Autodesk Fusion 360 part; units mm, degrees
(part 5 of 5)
  line L1149 (-30.3799, -38.9795, 1210.5243) -> (-23.832, -44.0828, 1211.5804) construction
  line L1150 (-23.832, -44.0828, 1211.5804) -> (-15.9786, -47.4967, 1212.6365) construction
  line L1151 (-15.9786, -47.4967, 1212.6365) -> (-7.7804, -48.8037, 1213.6926) construction
  line L1152 (-7.7804, -48.8037, 1213.6926) -> (0.4171, -50.1106, 1214.7486) construction
  line L1153 (0.4171, -50.1106, 1214.7486) -> (8.942, -49.3081, 1215.8046) construction
  line L1154 (8.942, -49.3081, 1215.8046) -> (16.7516, -46.4943, 1216.8606) construction
  line L1155 (16.7516, -46.4943, 1216.8606) -> (24.5605, -43.6808, 1217.9165) construction
  line L1156 (24.5605, -43.6808, 1217.9165) -> (31.6378, -38.8624, 1218.9725) construction
  line L1157 (31.6378, -38.8624, 1218.9725) -> (37.1178, -32.6282, 1220.0284) construction
  line L1158 (37.1178, -32.6282, 1220.0284) -> (42.5975, -26.3946, 1221.0842) construction
  line L1159 (42.5975, -26.3946, 1221.0842) -> (46.4686, -18.7588, 1222.1401) construction
  line L1160 (46.4686, -18.7588, 1222.1401) -> (48.2579, -10.6544, 1223.1959) construction
  line L1161 (48.2579, -10.6544, 1223.1959) -> (50.047, -2.5506, 1224.2516) construction
  line L1162 (50.047, -2.5506, 1224.2516) -> (49.7509, 6.0046, 1225.3074) construction
  line L1163 (49.7509, 6.0046, 1225.3074) -> (47.4058, 13.9653, 1226.3631) construction
  line L1164 (47.4058, 13.9653, 1226.3631) -> (45.0608, 21.9253, 1227.4188) construction
  line L1165 (45.0608, 21.9253, 1227.4188) -> (40.6721, 29.2741, 1228.4744) construction
  line L1166 (40.6721, 29.2741, 1228.4744) -> (34.7761, 35.1135, 1229.5301) construction
  line L1167 (34.7761, 35.1135, 1229.5301) -> (28.8806, 40.9524, 1230.5857) construction
  line L1168 (28.8806, 40.9524, 1230.5857) -> (21.4905, 45.2697, 1231.6412) construction
  line L1169 (21.4905, 45.2697, 1231.6412) -> (13.509, 47.5378, 1232.6968) construction
  line L1170 (13.509, 47.5378, 1232.6968) -> (5.528, 49.8058, 1233.7523) construction
  line L1171 (5.528, 49.8058, 1233.7523) -> (-3.0273, 50.0201, 1234.8078) construction
  line L1172 (-3.0273, 50.0201, 1234.8078) -> (-11.1118, 48.1546, 1235.8633) construction
  line L1173 (-11.1118, 48.1546, 1235.8633) -> (-19.1956, 46.2892, 1236.9187) construction
  line L1174 (-19.1956, 46.2892, 1236.9187) -> (-26.7915, 42.3483, 1237.9741) construction
  line L1175 (-26.7915, 42.3483, 1237.9741) -> (-32.9714, 36.8134, 1239.0295) construction
  line L1176 (-32.9714, 36.8134, 1239.0295) -> (-39.1508, 31.2788, 1240.0848) construction
  line L1177 (-39.1508, 31.2788, 1240.0848) -> (-43.9015, 24.1622, 1241.1401) construction
  line L1178 (-43.9015, 24.1622, 1241.1401) -> (-46.6431, 16.3327, 1242.1954) construction
  line L1179 (-46.6431, 16.3327, 1242.1954) -> (-49.3845, 8.5039, 1243.2507) construction
  line L1180 (-49.3845, 8.5039, 1243.2507) -> (-50.1113, -0.0211, 1244.3059) construction
  line L1181 (-50.1113, -0.0211, 1244.3059) -> (-48.7348, -8.201, 1245.3611) construction
  line L1182 (-48.7348, -8.201, 1245.3611) -> (-47.3584, -16.3803, 1246.4163) construction
  line L1183 (-47.3584, -16.3803, 1246.4163) -> (-43.8819, -24.1973, 1247.4714) construction
  line L1184 (-43.8819, -24.1973, 1247.4714) -> (-38.7299, -30.6974, 1248.5266) construction
  line L1185 (-38.7299, -30.6974, 1248.5266) -> (-33.5783, -37.1971, 1249.5817) construction
  line L1186 (-33.5783, -37.1971, 1249.5817) -> (-26.7622, -42.3663, 1250.6367) construction
  line L1187 (-26.7622, -42.3663, 1250.6367) -> (-19.114, -45.574, 1251.6918) construction
  line L1188 (-19.114, -45.574, 1251.6918) -> (-11.4664, -48.7815, 1252.7468) construction
  line L1189 (-11.4664, -48.7815, 1252.7468) -> (-3.0029, -50.0209, 1253.8018) construction
  line L1190 (-3.0029, -50.0209, 1253.8018) -> (5.2434, -49.1411, 1254.8568) construction
  line L1191 (5.2434, -49.1411, 1254.8568) -> (13.4889, -48.2613, 1255.9117) construction
  line L1192 (13.4889, -48.2613, 1255.9117) -> (21.4998, -45.2643, 1256.9666) construction
  line L1193 (21.4998, -45.2643, 1256.9666) -> (28.2982, -40.516, 1258.0215) construction
  line L1194 (28.2982, -40.516, 1258.0215) -> (35.096, -35.7681, 1259.0764) construction
  line L1195 (35.096, -35.7681, 1259.0764) -> (40.6672, -29.2792, 1260.1312) construction
  line L1196 (40.6672, -29.2792, 1260.1312) -> (44.3317, -21.8411, 1261.186) construction
  line L1197 (44.3317, -21.8411, 1261.186) -> (47.996, -14.4036, 1262.2408) construction
  line L1198 (47.996, -14.4036, 1262.2408) -> (49.7462, -6.0329, 1263.2955) construction
  line L1199 (49.7462, -6.0329, 1263.2955) -> (49.3688, 2.2497, 1264.3503) construction
  line L1200 (49.3688, 2.2497, 1264.3503) -> (48.9914, 10.5317, 1265.405) construction
  line L1201 (48.9914, 10.5317, 1265.405) -> (46.4874, 18.708, 1266.4597) construction
  line L1202 (46.4874, 18.708, 1266.4597) -> (42.1625, 25.781, 1267.5143) construction
  line L1203 (42.1625, 25.781, 1267.5143) -> (37.8378, 32.8536, 1268.5689) construction
  line L1204 (37.8378, 32.8536, 1268.5689) -> (31.7016, 38.8081, 1269.6235) construction
  line L1205 (31.7016, 38.8081, 1269.6235) -> (24.5023, 42.9182, 1270.6781) construction
  line L1206 (24.5023, 42.9182, 1270.6781) -> (17.3034, 47.0281, 1271.7327) construction
  line L1207 (17.3034, 47.0281, 1271.7327) -> (9.0569, 49.2851, 1272.7872) construction
  line L1208 (9.0569, 49.2851, 1272.7872) -> (0.7686, 49.414, 1273.8417) construction
  line L1209 (0.7686, 49.414, 1273.8417) -> (-7.5192, 49.5429, 1274.8962) construction
  line L1210 (-7.5192, 49.5429, 1274.8962) -> (-15.8313, 47.5438, 1275.9506) construction
  line L1211 (-15.8313, 47.5438, 1275.9506) -> (-23.1541, 43.6603, 1277.0051) construction
  line L1212 (-23.1541, 43.6603, 1277.0051) -> (-30.4764, 39.7772, 1278.0595) construction
  line L1213 (-30.4764, 39.7772, 1278.0595) -> (-36.7939, 34.0182, 1279.1138) construction
  line L1214 (-36.7939, 34.0182, 1279.1138) -> (-41.3365, 27.0857, 1280.1682) construction
  line L1215 (-41.3365, 27.0857, 1280.1682) -> (-45.8787, 20.1536, 1281.2225) construction
  line L1216 (-45.8787, 20.1536, 1281.2225) -> (-48.6365, 12.0628, 1282.2768) construction
  line L1217 (-48.6365, 12.0628, 1282.2768) -> (-49.2737, 3.7997, 1283.3311) construction
  line L1218 (-49.2737, 3.7997, 1283.3311) -> (-49.9109, -4.4628, 1284.3854) construction
  line L1219 (-49.9109, -4.4628, 1284.3854) -> (-48.4264, -12.8802, 1285.4396) construction
  line L1220 (-48.4264, -12.8802, 1285.4396) -> (-45.0012, -20.4263, 1286.4938) construction
  line L1221 (-45.0012, -20.4263, 1286.4938) -> (-41.5762, -27.9718, 1287.548) construction
  line L1222 (-41.5762, -27.9718, 1287.548) -> (-36.218, -34.6303, 1288.6022) construction
  line L1223 (-36.218, -34.6303, 1288.6022) -> (-29.5797, -39.5901, 1289.6563) construction
  line L1224 (-29.5797, -39.5901, 1289.6563) -> (-22.9419, -44.5496, 1290.7104) construction
  line L1225 (-22.9419, -44.5496, 1290.7104) -> (-15.0381, -47.8001, 1291.7645) construction
  line L1226 (-15.0381, -47.8001, 1291.7645) -> (-6.8317, -48.9455, 1292.8186) construction
  line L1227 (-6.8317, -48.9455, 1292.8186) -> (1.3741, -50.0909, 1293.8726) construction
  line L1228 (1.3741, -50.0909, 1293.8726) -> (9.8653, -49.129, 1294.9267) construction
  line L1229 (9.8653, -49.129, 1294.9267) -> (17.607, -46.1771, 1295.9807) construction
  line L1230 (17.607, -46.1771, 1295.9807) -> (25.3483, -43.2255, 1297.0346) construction
  line L1231 (25.3483, -43.2255, 1297.0346) -> (32.3239, -38.2903, 1298.0886) construction
  line L1232 (32.3239, -38.2903, 1298.0886) -> (37.6838, -31.9729, 1299.1426) construction
  line L1233 (37.6838, -31.9729, 1299.1426) -> (43.0435, -25.6559, 1300.1964) construction
  line L1234 (43.0435, -25.6559, 1300.1964) -> (46.7765, -17.9702, 1301.2503) construction
  line L1235 (46.7765, -17.9702, 1301.2503) -> (48.428, -9.8521, 1302.3042) construction
  line L1236 (48.428, -9.8521, 1302.3042) -> (50.0794, -1.7346, 1303.358) construction
  line L1237 (50.0794, -1.7346, 1303.358) -> (49.6462, 6.7981, 1304.4119) construction
  line L1238 (49.6462, 6.7981, 1304.4119) -> (47.181, 14.7066, 1305.4657) construction
  line L1239 (47.181, 14.7066, 1305.4657) -> (44.7161, 22.6147, 1306.5194) construction
  line L1240 (44.7161, 22.6147, 1306.5194) -> (40.2246, 29.8819, 1307.5732) construction
  line L1241 (40.2246, 29.8819, 1307.5732) -> (34.2538, 35.6232, 1308.6269) construction
  line L1242 (34.2538, 35.6232, 1308.6269) -> (28.2834, 41.3641, 1309.6806) construction
  line L1243 (28.2834, 41.3641, 1309.6806) -> (20.8463, 45.5672, 1310.7343) construction
  line L1244 (20.8463, 45.5672, 1310.7343) -> (12.8484, 47.7206, 1311.788) construction
  line L1245 (12.8484, 47.7206, 1311.788) -> (4.8509, 49.8738, 1312.8416) construction
  line L1246 (4.8509, 49.8738, 1312.8416) -> (-3.6905, 49.9731, 1313.8953) construction
  line L1247 (-3.6905, 49.9731, 1313.8953) -> (-11.7359, 48.0063, 1314.9489) construction
  line L1248 (-11.7359, 48.0063, 1314.9489) -> (-19.7807, 46.0396, 1316.0024) construction
  line L1249 (-19.7807, 46.0396, 1316.0024) -> (-27.3126, 42.0112, 1317.056) construction
  line L1250 (-27.3126, 42.0112, 1317.056) -> (-33.4145, 36.4117, 1318.1096) construction
  line L1251 (-33.4145, 36.4117, 1318.1096) -> (-39.5159, 30.8124, 1319.1631) construction
  line L1252 (-39.5159, 30.8124, 1319.1631) -> (-44.1747, 23.654, 1320.2166) construction
  line L1253 (-44.1747, 23.654, 1320.2166) -> (-46.8236, 15.8078, 1321.2701) construction
  line L1254 (-46.8236, 15.8078, 1321.2701) -> (-49.4724, 7.962, 1322.3235) construction
  line L1255 (-49.4724, 7.962, 1322.3235) -> (-50.1059, -0.5549, 1323.3769) construction
  line L1256 (-50.1059, -0.5549, 1323.3769) -> (-48.6471, -8.7061, 1324.4304) construction
  line L1257 (-48.6471, -8.7061, 1324.4304) -> (-47.1884, -16.8569, 1325.4837) construction
  line L1258 (-47.1884, -16.8569, 1325.4837) -> (-43.6407, -24.625, 1326.5371) construction
  line L1259 (-43.6407, -24.625, 1326.5371) -> (-38.4357, -31.0649, 1327.5905) construction
  line L1260 (-38.4357, -31.0649, 1327.5905) -> (-33.2311, -37.5045, 1328.6438) construction
  line L1261 (-33.2311, -37.5045, 1328.6438) -> (-26.3804, -42.6024, 1329.6971) construction
  line L1262 (-26.3804, -42.6024, 1329.6971) -> (-18.7174, -45.7383, 1330.7504) construction
  line L1263 (-18.7174, -45.7383, 1330.7504) -> (-11.0549, -48.8741, 1331.8037) construction
  line L1264 (-11.0549, -48.8741, 1331.8037) -> (-2.5962, -50.0414, 1332.8569) construction
  line L1265 (-2.5962, -50.0414, 1332.8569) -> (5.6293, -49.0983, 1333.9102) construction
  line L1266 (5.6293, -49.0983, 1333.9102) -> (13.8543, -48.1553, 1334.9634) construction
  line L1267 (13.8543, -48.1553, 1334.9634) -> (21.8289, -45.1041, 1336.0166) construction
  line L1268 (21.8289, -45.1041, 1336.0166) -> (28.5826, -40.3159, 1337.0698) construction
  line L1269 (28.5826, -40.3159, 1337.0698) -> (35.336, -35.5279, 1338.1229) construction
  line L1270 (35.336, -35.5279, 1338.1229) -> (40.8546, -29.0133, 1339.1761) construction
  line L1271 (40.8546, -29.0133, 1339.1761) -> (44.4669, -21.5645, 1340.2292) construction
  line L1272 (44.4669, -21.5645, 1340.2292) -> (48.079, -14.1162, 1341.2823) construction
  line L1273 (48.079, -14.1162, 1341.2823) -> (49.7776, -5.7495, 1342.3354) construction
  line L1274 (49.7776, -5.7495, 1342.3354) -> (49.3558, 2.5177, 1343.3884) construction
  line L1275 (49.3558, 2.5177, 1343.3884) -> (48.9341, 10.7846, 1344.4415) construction
  line L1276 (48.9341, 10.7846, 1344.4415) -> (46.3933, 18.9346, 1345.4945) construction
  line L1277 (46.3933, 18.9346, 1345.4945) -> (42.0424, 25.9764, 1346.5475) construction
  line L1278 (42.0424, 25.9764, 1346.5475) -> (37.6917, 33.0179, 1347.6005) construction
  line L1279 (37.6917, 33.0179, 1347.6005) -> (31.5403, 38.9365, 1348.6534) construction
  line L1280 (31.5403, 38.9365, 1348.6534) -> (24.3364, 43.0125, 1349.7064) construction
  line L1281 (24.3364, 43.0125, 1349.7064) -> (16.8312, 47.2589, 1350.8034) construction
  line L1282 (16.8312, 47.2589, 1350.8034) -> (8.1992, 49.4921, 1351.9004) construction
  line L1283 (8.1992, 49.4921, 1351.9004) -> (-0.4236, 49.4182, 1352.9974) construction
  line L1284 (-0.4236, 49.4182, 1352.9974) -> (-8.9118, 49.3454, 1354.0772) construction
  line L1285 (-8.9118, 49.3454, 1354.0772) -> (-17.3709, 47.0387, 1355.1571) construction
  line L1286 (-17.3709, 47.0387, 1355.1571) -> (-24.721, 42.7926, 1356.2369) construction
  line L1287 (-24.721, 42.7926, 1356.2369) -> (-31.9563, 38.6129, 1357.2999) construction
  line L1288 (-31.9563, 38.6129, 1357.2999) -> (-38.1014, 32.5643, 1358.3629) construction
  line L1289 (-38.1014, 32.5643, 1358.3629) -> (-42.3954, 25.3962, 1359.4259) construction
  line L1290 (-42.3954, 25.3962, 1359.4259) -> (-46.668, 18.2637, 1360.4836) construction
  line L1291 (-46.668, 18.2637, 1360.4836) -> (-49.0989, 10.0382, 1361.5413) construction
  line L1292 (-49.0989, 10.0382, 1361.5413) -> (-49.3897, 1.729, 1362.599) construction
  line L1293 (-49.3897, 1.729, 1362.599) -> (-49.6806, -6.5787, 1363.6565) construction
  line L1294 (-49.6806, -6.5787, 1363.6565) -> (-47.8316, -14.9523, 1364.714) construction
  line L1295 (-47.8316, -14.9523, 1364.714) -> (-44.0697, -22.3651, 1365.7715) construction
  line L1296 (-44.0697, -22.3651, 1365.7715) -> (-40.3085, -29.7764, 1366.8288) construction
  line L1297 (-40.3085, -29.7764, 1366.8288) -> (-34.6431, -36.2115, 1367.8861) construction
  line L1298 (-34.6431, -36.2115, 1367.8861) -> (-27.7679, -40.8813, 1368.9434) construction
  line L1299 (-27.7679, -40.8813, 1368.9434) -> (-20.8941, -45.5502, 1370.0005) construction
  line L1300 (-20.8941, -45.5502, 1370.0005) -> (-12.8257, -48.4447, 1371.0576) construction
  line L1301 (-12.8257, -48.4447, 1371.0576) -> (-4.5515, -49.21, 1372.1147) construction
  line L1302 (-4.5515, -49.21, 1372.1147) -> (3.7212, -49.9751, 1373.1716) construction
  line L1303 (3.7212, -49.9751, 1373.1716) -> (12.182, -48.6103, 1374.2285) construction
  line L1304 (12.182, -48.6103, 1374.2285) -> (19.7944, -45.2826, 1375.2853) construction
  line L1305 (19.7944, -45.2826, 1375.2853) -> (27.4055, -41.9556, 1376.342) construction
  line L1306 (27.4055, -41.9556, 1376.342) -> (34.1523, -36.6736, 1377.3987) construction
  line L1307 (34.1523, -36.6736, 1377.3987) -> (39.2087, -30.0835, 1378.4555) construction
  line L1308 (39.2087, -30.0835, 1378.4555) -> (44.2642, -23.4945, 1379.512) construction
  line L1309 (44.2642, -23.4945, 1379.512) -> (47.6191, -15.6119, 1380.5685) construction
  line L1310 (47.6191, -15.6119, 1380.5685) -> (48.8627, -7.4006, 1381.625) construction
  line L1311 (48.8627, -7.4006, 1381.625) -> (50.1062, 0.8092, 1382.6813) construction
  line L1312 (50.1062, 0.8092, 1382.6813) -> (49.2365, 9.3302, 1383.7376) construction
  line L1313 (49.2365, 9.3302, 1383.7376) -> (46.3601, 17.1195, 1384.7939) construction
  line L1314 (46.3601, 17.1195, 1384.7939) -> (43.4842, 24.9075, 1385.8501) construction
  line L1315 (43.4842, 24.9075, 1385.8501) -> (38.6084, 31.9476, 1386.9062) construction
  line L1316 (38.6084, 31.9476, 1386.9062) -> (32.3292, 37.3786, 1387.9624) construction
  line L1317 (32.3292, 37.3786, 1387.9624) -> (26.0511, 42.8086, 1389.0183) construction
  line L1318 (26.0511, 42.8086, 1389.0183) -> (18.3833, 46.6185, 1390.0743) construction
  line L1319 (18.3833, 46.6185, 1390.0743) -> (10.2637, 48.3424, 1391.1302) construction
  line L1320 (10.2637, 48.3424, 1391.1302) -> (2.1455, 50.0661, 1392.186) construction
  line L1321 (2.1455, 50.0661, 1392.186) -> (-6.4073, 49.7007, 1393.2418) construction
  line L1322 (-6.4073, 49.7007, 1393.2418) -> (-14.349, 47.291, 1394.2976) construction
  line L1323 (-14.349, 47.291, 1394.2976) -> (-22.2894, 44.8818, 1395.3532) construction
  line L1324 (-22.2894, 44.8818, 1395.3532) -> (-29.6021, 40.434, 1396.4088) construction
  line L1325 (-29.6021, 40.434, 1396.4088) -> (-35.3933, 34.4913, 1397.4644) construction
  line L1326 (-35.3933, 34.4913, 1397.4644) -> (-41.1836, 28.5496, 1398.5198) construction
  line L1327 (-41.1836, 28.5496, 1398.5198) -> (-45.4407, 21.126, 1399.5753) construction
  line L1328 (-45.4407, 21.126, 1399.5753) -> (-47.6446, 13.1275, 1400.6307) construction
  line L1329 (-47.6446, 13.1275, 1400.6307) -> (-49.848, 5.1303, 1401.686) construction
  line L1330 (-49.848, 5.1303, 1401.686) -> (-49.9942, -3.4246, 1402.7412) construction
  line L1331 (-49.9942, -3.4246, 1402.7412) -> (-48.0652, -11.4924, 1403.7965) construction
  line L1332 (-48.0652, -11.4924, 1403.7965) -> (-46.1365, -19.5589, 1404.8516) construction
  line L1333 (-46.1365, -19.5589, 1404.8516) -> (-42.1374, -27.1214, 1405.9067) construction
  line L1334 (-42.1374, -27.1214, 1405.9067) -> (-36.5561, -33.2564, 1406.9618) construction
  line L1335 (-36.5561, -33.2564, 1406.9618) -> (-30.9757, -39.3905, 1408.0168) construction
  line L1336 (-30.9757, -39.3905, 1408.0168) -> (-23.8255, -44.0846, 1409.0717) construction
  line L1337 (-23.8255, -44.0846, 1409.0717) -> (-15.9782, -46.7657, 1410.1266) construction
  line L1338 (-15.9782, -46.7657, 1410.1266) -> (-8.1321, -49.4465, 1411.1814) construction
  line L1339 (-8.1321, -49.4465, 1411.1814) -> (0.3942, -50.1092, 1412.2362) construction
  line L1340 (0.3942, -50.1092, 1412.2362) -> (8.5603, -48.673, 1413.291) construction
  line L1341 (8.5603, -48.673, 1413.291) -> (16.7251, -47.237, 1414.3456) construction
  line L1342 (16.7251, -47.237, 1414.3456) -> (24.5126, -43.7058, 1415.4003) construction
  line L1343 (24.5126, -43.7058, 1415.4003) -> (30.9727, -38.5101, 1416.4549) construction
  line L1344 (30.9727, -38.5101, 1416.4549) -> (37.4319, -33.3152, 1417.5094) construction
  line L1345 (37.4319, -33.3152, 1417.5094) -> (42.5503, -26.4673, 1418.5639) construction
  line L1346 (42.5503, -26.4673, 1418.5639) -> (45.7038, -18.8015, 1419.6184) construction
  line L1347 (45.7038, -18.8015, 1419.6184) -> (48.8569, -11.1369, 1420.6727) construction
  line L1348 (48.8569, -11.1369, 1420.6727) -> (50.0389, -2.6709, 1421.727) construction
  line L1349 (50.0389, -2.6709, 1421.727) -> (49.1058, 5.5643, 1422.7814) construction
  line L1350 (49.1058, 5.5643, 1422.7814) -> (48.1727, 13.7983, 1423.8356) construction
  line L1351 (48.1727, 13.7983, 1423.8356) -> (45.1271, 21.7842, 1424.8897) construction
  line L1352 (45.1271, 21.7842, 1424.8897) -> (40.3401, 28.5484, 1425.9439) construction
  line L1353 (40.3401, 28.5484, 1425.9439) -> (35.5538, 35.3117, 1426.998) construction
  line L1354 (35.5538, 35.3117, 1426.998) -> (29.0366, 40.8395, 1428.052) construction
  line L1355 (29.0366, 40.8395, 1428.052) -> (21.5829, 44.458, 1429.1061) construction
  line L1356 (21.5829, 44.458, 1429.1061) -> (14.1302, 48.0761, 1430.16) construction
  line L1357 (14.1302, 48.0761, 1430.16) -> (5.7568, 49.7778, 1431.2139) construction
  line L1358 (5.7568, 49.7778, 1431.2139) -> (-2.517, 49.3559, 1432.2678) construction
  line L1359 (-2.517, 49.3559, 1432.2678) -> (-10.7897, 48.934, 1433.3216) construction
  line L1360 (-10.7897, 48.934, 1433.3216) -> (-18.9455, 46.3899, 1434.3754) construction
  line L1361 (-18.9455, 46.3899, 1434.3754) -> (-25.9909, 42.0334, 1435.4292) construction
  line L1362 (-25.9909, 42.0334, 1435.4292) -> (-33.0354, 37.6775, 1436.4828) construction
  line L1363 (-33.0354, 37.6775, 1436.4828) -> (-38.955, 31.5189, 1437.5365) construction
  line L1364 (-38.955, 31.5189, 1437.5365) -> (-43.0288, 24.3076, 1438.5901) construction
  line L1365 (-43.0288, 24.3076, 1438.5901) -> (-47.1021, 17.0971, 1439.6436) construction
  line L1366 (-47.1021, 17.0971, 1439.6436) -> (-49.3215, 8.8493, 1440.6972) construction
  line L1367 (-49.3215, 8.8493, 1440.6972) -> (-49.4167, 0.5684, 1441.7507) construction
  line L1368 (-49.4167, 0.5684, 1441.7507) -> (-49.512, -7.7116, 1442.8041) construction
  line L1369 (-49.512, -7.7116, 1442.8041) -> (-47.4834, -16.0072, 1443.8575) construction
  line L1370 (-47.4834, -16.0072, 1443.8575) -> (-43.5779, -23.3089, 1444.9109) construction
  line L1371 (-43.5779, -23.3089, 1444.9109) -> (-39.6729, -30.6097, 1445.9642) construction
  line L1372 (-39.6729, -30.6097, 1445.9642) -> (-33.8996, -36.9013, 1447.0174) construction
  line L1373 (-33.8996, -36.9013, 1447.0174) -> (-26.9606, -41.4181, 1448.0707) construction
  line L1374 (-26.9606, -41.4181, 1448.0707) -> (-20.0224, -45.9345, 1449.1239) construction
  line L1375 (-20.0224, -45.9345, 1449.1239) -> (-11.9334, -48.6669, 1450.177) construction
  line L1376 (-11.9334, -48.6669, 1450.177) -> (-3.6777, -49.283, 1451.2302) construction
  line L1377 (-3.6777, -49.283, 1451.2302) -> (4.5771, -49.899, 1452.2833) construction
  line L1378 (4.5771, -49.899, 1452.2833) -> (12.9811, -48.3978, 1453.3363) construction
  line L1379 (12.9811, -48.3978, 1453.3363) -> (20.5122, -44.9621, 1454.3893) construction
  line L1380 (20.5122, -44.9621, 1454.3893) -> (28.4043, -41.3616, 1455.4929) construction
  line L1381 (28.4043, -41.3616, 1455.4929) -> (35.3172, -35.641, 1456.5964) construction
  line L1382 (35.3172, -35.641, 1456.5964) -> (40.3306, -28.5619, 1457.7) construction
  line L1383 (40.3306, -28.5619, 1457.7) -> (45.1873, -21.7039, 1458.769) construction
  line L1384 (45.1873, -21.7039, 1458.769) -> (48.2525, -13.5887, 1459.8381) construction
  line L1385 (48.2525, -13.5887, 1459.8381) -> (49.1422, -5.2323, 1460.9071) construction
  line L1386 (49.1422, -5.2323, 1460.9071) -> (50.0224, 3.0342, 1461.9647) construction
  line L1387 (50.0224, 3.0342, 1461.9647) -> (48.7726, 11.5186, 1463.0223) construction
  line L1388 (48.7726, 11.5186, 1463.0223) -> (45.5462, 19.1803, 1464.0798) construction
  line L1389 (45.5462, 19.1803, 1464.0798) -> (42.3209, 26.839, 1465.137) construction
  line L1390 (42.3209, 26.839, 1465.137) -> (37.1275, 33.6592, 1466.1942) construction
  line L1391 (37.1275, 33.6592, 1466.1942) -> (30.6023, 38.8051, 1467.2513) construction
  line L1392 (30.6023, 38.8051, 1467.2513) -> (24.0796, 43.949, 1468.3081) construction
  line L1393 (24.0796, 43.949, 1468.3081) -> (16.2401, 47.4089, 1469.3649) construction
  line L1394 (16.2401, 47.4089, 1469.3649) -> (8.0439, 48.761, 1470.4216) construction
  line L1395 (8.0439, 48.761, 1470.4216) -> (-0.1494, 50.1126, 1471.478) construction
  line L1396 (-0.1494, 50.1126, 1471.478) -> (-8.6816, 49.3551, 1472.5344) construction
  line L1397 (-8.6816, 49.3551, 1472.5344) -> (-16.5086, 46.5811, 1473.5908) construction
  line L1398 (-16.5086, 46.5811, 1473.5908) -> (-24.3328, 43.8082, 1474.6468) construction
  line L1399 (-24.3328, 43.8082, 1474.6468) -> (-31.4357, 39.0261, 1475.7028) construction
  line L1400 (-31.4357, 39.0261, 1475.7028) -> (-36.9485, 32.8199, 1476.7589) construction
  line L1401 (-36.9485, 32.8199, 1476.7589) -> (-42.4594, 26.6157, 1477.8145) construction
  line L1402 (-42.4594, 26.6157, 1477.8145) -> (-46.3696, 19.0014, 1478.8702) construction
  line L1403 (-46.3696, 19.0014, 1478.8702) -> (-48.2012, 10.9078, 1479.9259) construction
  line L1404 (-48.2012, 10.9078, 1479.9259) -> (-50.0322, 2.8167, 1480.9812) construction
  line L1405 (-50.0322, 2.8167, 1480.9812) -> (-49.782, -5.7363, 1482.0365) construction
  line L1406 (-49.782, -5.7363, 1482.0365) -> (-47.4812, -13.7065, 1483.0918) construction
  line L1407 (-47.4812, -13.7065, 1483.0918) -> (-45.1812, -21.6742, 1484.1468) construction
  line L1408 (-45.1812, -21.6742, 1484.1468) -> (-40.8367, -29.0427, 1485.2018) construction
  line L1409 (-40.8367, -29.0427, 1485.2018) -> (-34.9781, -34.9123, 1486.2568) construction
  line L1410 (-34.9781, -34.9123, 1486.2568) -> (-29.1213, -40.7802, 1487.3115) construction
  line L1411 (-29.1213, -40.7802, 1487.3115) -> (-21.7637, -45.1377, 1488.3662) construction
  line L1412 (-21.7637, -45.1377, 1488.3662) -> (-13.803, -47.4533, 1489.4209) construction
  line L1413 (-13.803, -47.4533, 1489.4209) -> (-5.8446, -49.7682, 1490.4753) construction
  line L1414 (-5.8446, -49.7682, 1490.4753) -> (2.6998, -50.0374, 1491.5297) construction
  line L1415 (2.6998, -50.0374, 1491.5297) -> (10.7882, -48.2281, 1492.584) construction
  line L1416 (10.7882, -48.2281, 1492.584) -> (18.8743, -46.4193, 1493.6381) construction
  line L1417 (18.8743, -46.4193, 1493.6381) -> (26.4877, -42.537, 1494.6922) construction
  line L1418 (26.4877, -42.537, 1494.6922) -> (32.7004, -37.0543, 1495.7463) construction
  line L1419 (32.7004, -37.0543, 1495.7463) -> (38.9115, -31.573, 1496.8002) construction
  line L1420 (38.9115, -31.573, 1496.8002) -> (43.7096, -24.5037, 1497.854) construction
  line L1421 (43.7096, -24.5037, 1497.854) -> (46.5101, -16.7076, 1498.9078) construction
  line L1422 (46.5101, -16.7076, 1498.9078) -> (49.31, -8.9134, 1499.9614) construction
  line L1423 (49.31, -8.9134, 1499.9614) -> (50.1075, -0.4092, 1501.015) construction
  line L1424 (50.1075, -0.4092, 1501.015) -> (48.8054, 7.7697, 1502.0685) construction
  line L1425 (48.8054, 7.7697, 1502.0685) -> (47.5037, 15.9466, 1503.1219) construction
  line L1426 (47.5037, 15.9466, 1503.1219) -> (44.1062, 23.781, 1504.1752) construction
  line L1427 (44.1062, 23.781, 1504.1752) -> (39.0264, 30.3195, 1505.2285) construction
  line L1428 (39.0264, 30.3195, 1505.2285) -> (33.9478, 36.8566, 1506.2816) construction
  line L1429 (33.9478, 36.8566, 1506.2816) -> (27.1983, 42.0846, 1507.3347) construction
  line L1430 (27.1983, 42.0846, 1507.3347) -> (19.5991, 45.3675, 1508.3877) construction
  line L1431 (19.5991, 45.3675, 1508.3877) -> (11.7904, 48.7409, 1509.4699) construction
  line L1432 (11.7904, 48.7409, 1509.4699) -> (3.1011, 50.0507, 1510.552) construction
  line L1433 (3.1011, 50.0507, 1510.552) -> (-5.355, 49.129, 1511.6341) construction
  line L1434 (-5.355, 49.129, 1511.6341) -> (-13.6173, 48.2284, 1512.6914) construction
  line L1435 (-13.6173, 48.2284, 1512.6914) -> (-21.6389, 45.2014, 1513.7487) construction
  line L1436 (-21.6389, 45.2014, 1513.7487) -> (-28.4364, 40.4191, 1514.806) construction
  line L1437 (-28.4364, 40.4191, 1514.806) -> (-35.2289, 35.6404, 1515.8625) construction
  line L1438 (-35.2289, 35.6404, 1515.8625) -> (-40.7846, 29.1192, 1516.919) construction
  line L1439 (-40.7846, 29.1192, 1516.919) -> (-44.4235, 21.6538, 1517.9756) construction
  line L1440 (-44.4235, 21.6538, 1517.9756) -> (-48.06, 14.1935, 1519.0314) construction
  line L1441 (-48.06, 14.1935, 1519.0314) -> (-49.7745, 5.8063, 1520.0872) construction
  line L1442 (-49.7745, 5.8063, 1520.0872) -> (-49.3576, -2.4825, 1521.1429) construction
  line L1443 (-49.3576, -2.4825, 1521.1429) -> (-48.941, -10.766, 1522.1981) construction
  line L1444 (-48.941, -10.766, 1522.1981) -> (-46.3965, -18.9338, 1523.2532) construction
  line L1445 (-46.3965, -18.9338, 1523.2532) -> (-42.035, -25.9883, 1524.3083) construction
  line L1446 (-42.035, -25.9883, 1524.3083) -> (-37.6761, -33.0388, 1525.3628) construction
  line L1447 (-37.6761, -33.0388, 1525.3628) -> (-31.5114, -38.9625, 1526.4173) construction
  line L1448 (-31.5114, -38.9625, 1526.4173) -> (-24.2929, -43.0371, 1527.4718) construction
  line L1449 (-24.2929, -43.0371, 1527.4718) -> (-17.0783, -47.1095, 1528.5257) construction
  line L1450 (-17.0783, -47.1095, 1528.5257) -> (-8.8262, -49.3262, 1529.5796) construction
  line L1451 (-8.8262, -49.3262, 1529.5796) -> (-0.5421, -49.417, 1530.6335) construction
  line L1452 (-0.5421, -49.417, 1530.6335) -> (7.738, -49.5079, 1531.6869) construction
  line L1453 (7.738, -49.5079, 1531.6869) -> (16.0326, -47.4748, 1532.7404) construction
  line L1454 (16.0326, -47.4748, 1532.7404) -> (23.3322, -43.5654, 1533.7938) construction
  line L1455 (23.3322, -43.5654, 1533.7938) -> (30.9937, -39.4621, 1534.8994) construction
  line L1456 (30.9937, -39.4621, 1534.8994) -> (37.5387, -33.2975, 1536.005) construction
  line L1457 (37.5387, -33.2975, 1536.005) -> (42.0926, -25.895, 1537.1107) construction
  line L1458 (42.0926, -25.895, 1537.1107) -> (46.4452, -18.8198, 1538.1674) construction
  line L1459 (46.4452, -18.8198, 1538.1674) -> (48.9724, -10.6321, 1539.2242) construction
  line L1460 (48.9724, -10.6321, 1539.2242) -> (49.3648, -2.3346, 1540.2809) construction
  line L1461 (49.3648, -2.3346, 1540.2809) -> (49.7567, 5.9516, 1541.3362) construction
  line L1462 (49.7567, 5.9516, 1541.3362) -> (48.0188, 14.3298, 1542.3915) construction
  line L1463 (48.0188, 14.3298, 1542.3915) -> (44.3635, 21.7765, 1543.4468) construction
  line L1464 (44.3635, 21.7765, 1543.4468) -> (40.7124, 29.2145, 1544.5009) construction
  line L1465 (40.7124, 29.2145, 1544.5009) -> (35.1561, 35.7077, 1545.555) construction
  line L1466 (35.1561, 35.7077, 1545.555) -> (28.3718, 40.4646, 1546.6091) construction
  line L1467 (28.3718, 40.4646, 1546.6091) -> (21.5939, 45.2169, 1547.6621) construction
  line L1468 (21.5939, 45.2169, 1547.6621) -> (13.6046, 48.2263, 1548.7152) construction
  line L1469 (13.6046, 48.2263, 1548.7152) -> (5.3758, 49.1267, 1549.7683) construction
  line L1470 (5.3758, 49.1267, 1549.7683) -> (-2.874, 50.0295, 1550.824) construction
  line L1471 (-2.874, 50.0295, 1550.824) -> (-11.3473, 48.8104, 1551.8798) construction
  line L1472 (-11.3473, 48.8104, 1551.8798) -> (-19.008, 45.6183, 1552.9356) construction
  line L1473 (-19.008, 45.6183, 1552.9356) -> (-26.6514, 42.4335, 1553.989) construction
  line L1474 (-26.6514, 42.4335, 1553.989) -> (-33.4699, 37.2916, 1555.0423) construction
  line L1475 (-33.4699, 37.2916, 1555.0423) -> (-38.6336, 30.8185, 1556.0957) construction
  line L1476 (-38.6336, 30.8185, 1556.0957) -> (-43.8008, 24.341, 1557.1498) construction
  line L1477 (-43.8008, 24.341, 1557.1498) -> (-47.3, 16.5441, 1558.2039) construction
  line L1478 (-47.3, 16.5441, 1558.2039) -> (-48.7047, 8.378, 1559.258) construction
  line L1479 (-48.7047, 8.378, 1559.258) -> (-49.1804, 5.6124, 1559.615) construction
  line L1480 (-49.1804, 5.6124, 1559.615) -> (-49.42, 2.8062, 1559.972) construction
  line L1481 (-49.42, 2.8062, 1559.972) -> (-49.42, 0, 1560.329) construction
  spline S1 degree 5 poles (49.42, 0, -20) (49.42, 0, -18.5646) (49.4177, 0.2115, -15.7899) (49.4072, 1.1626, -11.9166) (49.3448, 3.5363, -7.2986) (48.9553, 7.8197, -2.4796) (48.1121, 12.0242, 0.3973) (46.9949, 15.5703, 1.8031) (45.9973, 18.1153, 2.3586) (45.4352, 19.4331, 2.5409) knots 0 0 0 0 0 0 0.2 0.4 0.6 0.8 1 1 1 1 1 1
  dimension "d16" = 20
  dimension "d17" = 40
pipe "Leitung2" add diameter 6 path "Skizze7" along L1 S1 S0 separate body makes body 2
hidden bodies 1
equation "d6 = ( 39.502 * 39.5 ) * 1 mm"
equation "d10 = ( 39.303 * 39.502 ) * 1 mm"
named bodies: "Sketch Spiral", "Copper Wire"
